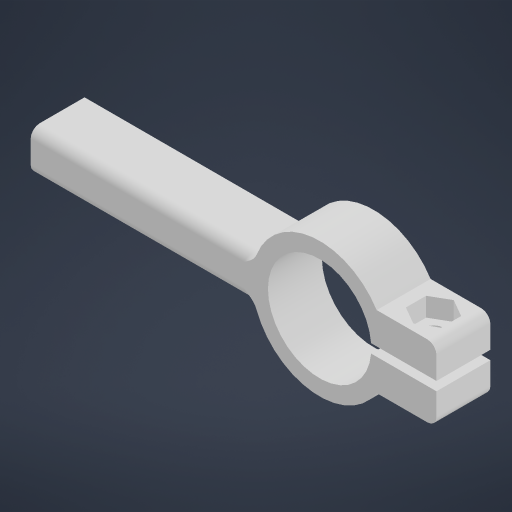
# Autodesk Inventor part: Clasp
Saved by Autodesk Inventor 2024.1 (Build 281209000, 209)
## iProperties
Created: 2023-09-06
Part Number: Clasp
Material: Generic
Document SubType Name: Modeling
Designer: User
Density: 1 g/cm^3
Appearance: Default
Author: User
Autodesk Inventor part; units mm, degrees
ref_plane "YZ Plane" through (0, 0, 0) normal (1, 0, 0) x (0, 1, 0)
ref_plane "XZ Plane" through (0, 0, 0) normal (0, 1, 0) x (-1, 0, 0)
ref_plane "XY Plane" through (0, 0, 0) normal (0, 0, 1) x (1, 0, 0)
sketch "Sketch1" plane through (0, 0, 0) normal (0, 0, 1) x (1, 0, 0)
  circle A0 centre (0, 0) radius 11.5
  circle A1 centre (0, 0) radius 15
  line L0 (26, 8) -> (11.5, 8)
  line L1 (11.5, 8) -> (11.5, -8)
  line L2 (11.5, -8) -> (26, -8)
  line L3 (26, -8) -> (26, 8)
  line L4 (-64.309, 4.5) -> (-12, 4.5)
  line L5 (-12, 4.5) -> (-12, -4.5)
  line L6 (-12, -4.5) -> (-64.309, -4.5)
  line L7 (-64.309, -4.5) -> (-64.309, 4.5)
  point P0 (12.6886, 8)
  point P1 (12.6886, -8)
  point P2 (-14.3091, -4.5)
  point P3 (-14.3091, 4.5)
  dimension "d0" = 23
  dimension "d1" = 30
  dimension "d10" = 14.5
  dimension "d11" = 16
  dimension "d45" = 52.309
  dimension "d46" = 9
  constraints: 16 end point, 4 parallel, 2 centre point, 2 coincident, 2 horizontal, 2 perpendicular, 1 other
  measures "d0" diameter of A0
  measures "d1" diameter of A1
  measures "d10" distance of L2.end L1.end
  measures "d11" distance of L1.end L0.end
  measures "d45" distance of L5.end L6.end
  measures "d46" distance of L4.end L5.end
extrude "Extrusion1" add sketch "Sketch1" along normal blind 12
sketch "Sketch2" plane through (0, 0, 12) normal (0, 0, 1) x (1, 0, 0)
  circle A0 centre (0, 0) radius 11.5 projected
  line L0 (26, -8) -> (26, 8) projected
  line L1 (26, 0) -> (11.3, 0)
  line L2 (11.3, 0) -> (11.3, 1)
  line L3 (11.3, 1) -> (26, 1)
  line L4 (26, 1) -> (26, 0)
  line L5 (26, 0) -> (11.3, 0)
  line L6 (11.3, 0) -> (11.3, -1)
  line L7 (11.3, -1) -> (26, -1)
  line L8 (26, -1) -> (26, 0)
  point P0 (11.4564, 1)
  point P1 (11.4564, -1)
  dimension "d20" = 14.7
  dimension "d21" = 1
  dimension "d22" = 1
  constraints: 16 end point, 4 parallel, 2 horizontal, 2 perpendicular, 1 midpoint, 1 point on line
  measures "d20" distance of L2.end L3.end
  measures "d21" distance of L1.end L2.end
  measures "d22" distance of L6.end L5.end
extrude "Extrusion2" cut sketch "Sketch2" against normal blind 12 contours L1 L2 L3 A0 | L1 L0 L7 A0 | A0 L3 L0 L1 | A0 L7 L6 L1
sketch "Sketch3" plane through (12.6886, -8, 0) normal (0, -1, 0) x (1, 0, 0)
  line L0 (0, 0) -> (0, 12) projected
  line L1 (0, 0) -> (6.6555, 0)
  line L2 (6.6555, 0) -> (6.6555, 6)
  line L3 (6.6555, 6) -> (0, 6)
  line L4 (0, 6) -> (0, 0)
  point P0 (-12.6886, 0)
  dimension "d25" = 6.6555
  dimension "d26" = 6
  constraints: 8 end point, 2 parallel, 1 coincident, 1 horizontal, 1 perpendicular
  measures "d25" distance of L3.end L2.end
  measures "d26" distance of L2.end L1.end
hole "Hole1" at (19.3441, -8, 6) direction (0, 1, 0) diameter 4.5 depth 16 counterbore diameter 8.5 counterbore depth 3.5
sketch "Sketch4" plane through (12.6886, 8, 0) normal (0, 1, 0) x (1, 0, 0)
  line L0 (13.3114, 0) -> (0, 0) projected
  line L1 (0, 0) -> (6.6555, 0)
  line L2 (6.6555, 0) -> (6.6555, -6)
  line L3 (6.6555, -6) -> (0, -6)
  line L4 (0, -6) -> (0, 0)
  line L5 (6.6555, -6) -> (6.6555, -10.5)
  line L6 (6.6555, -6) -> (11.1555, -6) construction
  line L7 (6.6555, -10.5) -> (2.7584, -8.25)
  line L8 (2.7584, -8.25) -> (2.7584, -3.75)
  line L9 (2.7584, -3.75) -> (6.6555, -1.5)
  line L10 (6.6555, -1.5) -> (10.5526, -3.75)
  line L11 (10.5526, -3.75) -> (10.5526, -8.25)
  line L12 (10.5526, -8.25) -> (6.6555, -10.5)
  point P0 (-12.6886, 0)
  dimension "d51" = 6.6555
  dimension "d52" = 6
  dimension "d53" = 4.5
  dimension "d54" = 90
  constraints: 24 end point, 2 coincident, 2 horizontal, 2 parallel, 2 perpendicular, 1 vertical, 13 other
  measures "d51" distance of L2.end L3.end
  measures "d52" distance of L1.end L2.end
  measures "d53" distance of L5.start L5.end
  measures "d54" angle of L5 L6
extrude "Extrusion3" cut sketch "Sketch4" against normal blind 4.2 contours L10 L11 L12 L5 L2 | L2 L3 L8 L9 | L5 L7 L8 L3
fillet "Fillet1" radius 2 2 edges at (-39.309, 4.5, 12) (-39.309, -4.5, 12)
fillet "Fillet2" radius 2 4 edges at (-14.3091, -4.5, 5) (-14.4562, -4.0024, 11.3202) (-14.3091, 4.5, 5) (-14.4562, 4.0024, 11.3201)
fillet "Fillet3" radius 2 2 edges at (26, -8, 6) (26, 8, 6)
body "Solid1"
